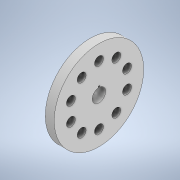
# Autodesk Inventor part: Circular Pattern
Saved by Autodesk Inventor 2020 (Build 240168000, 168)
## iProperties
Created: 2020-01-30
Part Number: Circular Pattern
Material: Generic
Document SubType Name: Modeling
Designer: cks4a449
Density: 1 g/cm^3
Appearance: Default
Author: cks4a449
Autodesk Inventor part; units mm, degrees
ref_plane "YZ Plane" through (0, 0, 0) normal (1, 0, 0) x (0, 1, 0)
ref_plane "XZ Plane" through (0, 0, 0) normal (0, 1, 0) x (-1, 0, 0)
ref_plane "XY Plane" through (0, 0, 0) normal (0, 0, 1) x (1, 0, 0)
sketch "Sketch1" plane through (0, 0, 0) normal (0, 0, 1) x (1, 0, 0)
  line L0 (0, 0) -> (15.2339, 0)
  line L1 (15.2339, 0) -> (15.2339, 9.525)
  line L2 (15.2339, 9.525) -> (40.6339, 9.525)
  line L3 (40.6339, 9.525) -> (40.6339, 63.5)
  line L4 (40.6339, 63.5) -> (27.9339, 63.5)
  line L5 (27.9339, 63.5) -> (27.9339, 25.4)
  line L6 (27.9339, 25.4) -> (15.2339, 25.4)
  line L7 (15.2339, 25.4) -> (15.2339, 9.525)
  dimension "d0" = 9.525
  dimension "d1" = 12.7
  dimension "d2" = 25.4
  dimension "d3" = 63.5
  dimension "d4" = 25.4
  constraints: 16 end point, 6 perpendicular, 1 horizontal, 1 point on line, 1 vertical
  measures "d0" distance of L0.end L1.end
  measures "d1" distance of L3.end L4.end
  measures "d2" distance of L1.end L2.end
  measures "d3" distance from line of L0 L3.end
  measures "d4" distance between parallel lines of L0 L6
revolve "Revolution1" add sketch "Sketch1" angle 360 about axis through (0, 0, 0) along (1, 0, 0)
sketch "Sketch2" plane through (15.2339, 0, 0) normal (-1, 0, 0) x (0, 0, 1)
  line L0 (-1.27, 8.2149) -> (1.27, 8.2149)
  line L1 (1.27, 8.2149) -> (1.27, 11.43)
  line L2 (1.27, 11.43) -> (-1.27, 11.43)
  line L3 (-1.27, 11.43) -> (-1.27, 8.2149)
  line L4 (-1.27, 8.2149) -> (1.27, 11.43) construction
  line L5 (1.27, 8.2149) -> (-1.27, 11.43) construction
  point P0 (0, 0)
  point P1 (0, 9.8225)
  dimension "d6" = 11.43
  dimension "d7" = 1.27
  dimension "d8" = 1.27
  constraints: 12 end point, 2 midpoint, 2 parallel, 1 horizontal, 1 perpendicular
  measures "d6" distance from line of L2 point (0, 0)
  measures "d7" distance from line of point (0, 0) L1
  measures "d8" distance from line of point (0, 0) L3
extrude "Extrusion1" cut sketch "Sketch2" against normal through all
sketch "Sketch3" plane through (27.9339, 0, 0) normal (-1, 0, 0) x (0, 0, 1)
  point P0 (0, 0)
  point P1 (0, 41.91)
  point P2 (-24.6341, 33.9059)
  point P3 (-39.8588, 12.9509)
  point P4 (-39.8588, -12.9509)
  point P5 (-24.6341, -33.9059)
  point P6 (0, -41.91)
  point P7 (24.6341, -33.9059)
  point P8 (39.8588, -12.9509)
  point P9 (39.8588, 12.9509)
  point P10 (24.6341, 33.9059)
  dimension "d11" = 41.91
  dimension "d12" = 0
  dimension "d15" = 360
  constraints: 11 other
  measures "d11" distance of point (0, 0) point (0, 41.91)
  measures "d12" horizontal distance of point (0, 0) point (0, 41.91)
hole "Hole1" at (27.9339, 41.91, 0) at (27.9339, 33.9059, -24.6341) at (27.9339, 12.9509, -39.8588) at (27.9339, -12.9509, -39.8588) at (27.9339, -33.9059, -24.6341) at (27.9339, -41.91, 0) at (27.9339, -33.9059, 24.6341) at (27.9339, -12.9509, 39.8588) at (27.9339, 12.9509, 39.8588) at (27.9339, 33.9059, 24.6341) direction (1, 0, 0) diameter 12.7 end through all clearance for "Hex Head Bolt" size "1/2" standard "Ansi Unified Screw Threads"
body "Solid1"
